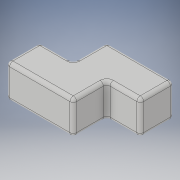
# Autodesk Inventor part: tetris_object_cca20_chamfered
Saved by Autodesk Inventor 2017 (Build 210142000, 142)
## iProperties
Part Number: tetris_object_cca20_chamfered
Material: Všeobecné
Document SubType Name: Modeling
Designer: TM
Density: 1 g/cm^3
Appearance: Výchozí
Author: TM
Autodesk Inventor part; units mm, degrees
ref_plane "YZ Plane" through (0, 0, 0) normal (1, 0, 0) x (0, 1, 0)
ref_plane "XZ Plane" through (0, 0, 0) normal (0, 1, 0) x (-1, 0, 0)
ref_plane "XY Plane" through (0, 0, 0) normal (0, 0, 1) x (1, 0, 0)
sketch "Náčrt1" plane through (0, 0, 0) normal (0, 0, 1) x (1, 0, 0)
  line L0 (0, 0) -> (0.025, 0) construction
  line L1 (0.025, 0) -> (0.025, 0) construction
  line L2 (0.025, 0) -> (0.075, 0)
  line L3 (0.075, 0) -> (0.075, 0.05)
  line L4 (0.075, 0.05) -> (-0.025, 0.05)
  line L5 (-0.025, 0.05) -> (-0.025, 0)
  line L6 (-0.025, 0) -> (-0.075, 0)
  line L7 (-0.075, 0) -> (-0.075, -0.05)
  line L8 (-0.075, -0.05) -> (0.025, -0.05)
  line L9 (0.025, -0.05) -> (0.025, 0)
  dimension "d14" = 0.025
  dimension "d15" = 0
  dimension "d16" = 0.05
  dimension "d17" = 0.05
  dimension "d18" = 0.1
  dimension "d19" = 0.05
  dimension "d20" = 0.05
  dimension "d21" = 0.05
  dimension "d22" = 0.1
  dimension "d23" = 0.05
  constraints: 20 end point, 6 perpendicular, 2 horizontal, 2 vertical, 1 point on line
  measures "d14" distance of L0.start L0.end
  measures "d15" distance of L0.end L1.end
  measures "d16" distance of L1.end L2.end
  measures "d17" distance of L2.end L3.end
  measures "d18" distance of L3.end L4.end
  measures "d19" distance of L4.end L5.end
  measures "d20" distance of L5.end L6.end
  measures "d21" distance of L6.end L7.end
  measures "d22" distance of L7.end L8.end
  measures "d23" distance of L8.end L1.end
extrude "Vysunutí1" add sketch "Náčrt1" along normal mid plane 0.05
fillet "Zaoblení1" radius 0.005 22 edges at (0.025, -0.05, 0) (0.025, -0.025, 0.025) (0.025, -0.025, -0.025) (-0.075, -0.05, 0) (-0.025, -0.05, 0.025) (-0.025, -0.05, -0.025) (0.05, 0, 0.025) (0.075, 0, 0) (0.05, 0, -0.025) (-0.075, -0.025, 0.025) (-0.05, 0, 0.025) (-0.025, 0.025, 0.025) (0.025, 0.05, 0.025) (0.075, 0.025, 0.025) (-0.075, 0, 0) (-0.075, -0.025, -0.025) (0.075, 0.05, 0) (0.075, 0.025, -0.025) (-0.05, 0, -0.025) (-0.025, 0.025, -0.025) (0.025, 0.05, -0.025) (-0.025, 0.05, 0)
fillet "Zaoblení1" radius 0.005 2 edges at (0.025, 0, 0) (-0.025, 0, 0)
equation "\"d16\" = 2 * d14"
equation "\"d17\" = d16"
equation "\"d18\" = 2 * d16"
equation "\"d19\" = d16"
equation "\"d20\" = d16"
equation "\"d21\" = d16"
equation "\"d10\" = d16"
equation "\"d12\" = 0.1 * d16"
equation "\"d13\" = 0.1 * d16"
